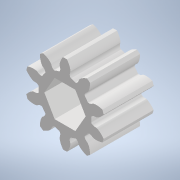
# Autodesk Inventor part: engranaje10
Saved by Autodesk Inventor 2022 (Build 260153000, 153)
## iProperties
Created: 2022-03-10
Part Number: engranaje10
Material: Generic
Document SubType Name: Modeling
Designer: katha
Density: 1 g/cm^3
Appearance: Default
Author: katha
Autodesk Inventor part; units mm, degrees
(part 1 of 2)
ref_plane "YZ Plane" through (0, 0, 0) normal (1, 0, 0) x (0, 1, 0)
ref_plane "XZ Plane" through (0, 0, 0) normal (0, 1, 0) x (-1, 0, 0)
ref_plane "XY Plane" through (0, 0, 0) normal (0, 0, 1) x (1, 0, 0)
sketch "Sketch1" plane through (0, 0, 0) normal (0, 0, 1) x (1, 0, 0)
  circle A0 centre (25, 0) radius 2
  circle A1 centre (25, 0) radius 2
  line L0 (21.2429, -4.5485) -> (21.2518, -4.404)
  line L1 (21.2518, -4.404) -> (21.266, -4.2669)
  line L2 (21.266, -4.2669) -> (21.2847, -4.1394)
  line L3 (21.2847, -4.1394) -> (21.3072, -4.0209)
  line L4 (21.3072, -4.0209) -> (21.3326, -3.9121)
  line L5 (21.3326, -3.9121) -> (21.3609, -3.8103)
  line L6 (21.3609, -3.8103) -> (21.3897, -3.7211)
  line L7 (21.3897, -3.7211) -> (21.4209, -3.6371)
  line L8 (21.4209, -3.6371) -> (21.4808, -3.5016)
  line L9 (21.4808, -3.5016) -> (21.5378, -3.3972)
  line L10 (21.5378, -3.3972) -> (21.5846, -3.3262)
  line L11 (21.5846, -3.3262) -> (21.6076, -3.2964)
  line L12 (21.6076, -3.2964) -> (21.7008, -3.2317)
  line L13 (21.7008, -3.2317) -> (21.7827, -3.1653)
  line L14 (21.7827, -3.1653) -> (21.8534, -3.098)
  line L15 (21.8534, -3.098) -> (21.9129, -3.0308)
  line L16 (21.9129, -3.0308) -> (21.9613, -2.9643)
  line L17 (21.9613, -2.9643) -> (21.9989, -2.8995)
  line L18 (21.9989, -2.8995) -> (22.026, -2.837)
  line L19 (22.026, -2.837) -> (22.0427, -2.7777)
  line L20 (22.0427, -2.7777) -> (22.0493, -2.7222)
  line L21 (22.0493, -2.7222) -> (22.0464, -2.6714)
  line L22 (22.0464, -2.6714) -> (22.0342, -2.626)
  line L23 (22.0342, -2.626) -> (22.0067, -2.5776)
  line L24 (22.0067, -2.5776) -> (21.911, -2.4618)
  line L25 (21.911, -2.4618) -> (21.8044, -2.3218)
  line L26 (21.8044, -2.3218) -> (21.7042, -2.1772)
  line L27 (21.7042, -2.1772) -> (21.6236, -2.0503)
  line L28 (21.6236, -2.0503) -> (21.5861, -2.0092)
  line L29 (21.5861, -2.0092) -> (21.5466, -1.9836)
  line L30 (21.5466, -1.9836) -> (21.4992, -1.9651)
  line L31 (21.4992, -1.9651) -> (21.4444, -1.9544)
  line L32 (21.4444, -1.9544) -> (21.3828, -1.9519)
  line L33 (21.3828, -1.9519) -> (21.3151, -1.9583)
  line L34 (21.3151, -1.9583) -> (21.2418, -1.974)
  line L35 (21.2418, -1.974) -> (21.1636, -1.9996)
  line L36 (21.1636, -1.9996) -> (21.0812, -2.0354)
  line L37 (21.0812, -2.0354) -> (20.9955, -2.0818)
  line L38 (20.9955, -2.0818) -> (20.907, -2.1392)
  line L39 (20.907, -2.1392) -> (20.8167, -2.2078)
  line L40 (20.8167, -2.2078) -> (20.7812, -2.2206)
  line L41 (20.7812, -2.2206) -> (20.6993, -2.2432)
  line L42 (20.6993, -2.2432) -> (20.5824, -2.2651)
  line L43 (20.5824, -2.2651) -> (20.4349, -2.2802)
  line L44 (20.4349, -2.2802) -> (20.3454, -2.2839)
  line L45 (20.3454, -2.2839) -> (20.2517, -2.2838)
  line L46 (20.2517, -2.2838) -> (20.1462, -2.2793)
  line L47 (20.1462, -2.2793) -> (20.0348, -2.2698)
  line L48 (20.0348, -2.2698) -> (19.9152, -2.2546)
  line L49 (19.9152, -2.2546) -> (19.7881, -2.2329)
  line L50 (19.7881, -2.2329) -> (19.6534, -2.2041)
  line L51 (19.6534, -2.2041) -> (19.5132, -2.1679)
  line L52 (19.5132, -2.1679) -> (19.3913, -2.1313)
  arc A2 (19.2098, -1.5727) -> (19.3913, -2.1313) centre (25, 0) ccw
  line L53 (19.2098, -1.5727) -> (19.2869, -1.4714)
  line L54 (19.2869, -1.4714) -> (19.379, -1.3597)
  line L55 (19.379, -1.3597) -> (19.4711, -1.2572)
  line L56 (19.4711, -1.2572) -> (19.5612, -1.165)
  line L57 (19.5612, -1.165) -> (19.649, -1.0823)
  line L58 (19.649, -1.0823) -> (19.7335, -1.0092)
  line L59 (19.7335, -1.0092) -> (19.8162, -0.9435)
  line L60 (19.8162, -0.9435) -> (19.892, -0.8884)
  line L61 (19.892, -0.8884) -> (19.9665, -0.8387)
  line L62 (19.9665, -0.8387) -> (20.0947, -0.7643)
  line L63 (20.0947, -0.7643) -> (20.2022, -0.7133)
  line L64 (20.2022, -0.7133) -> (20.2818, -0.6834)
  line L65 (20.2818, -0.6834) -> (20.3179, -0.6728)
  line L66 (20.3179, -0.6728) -> (20.4313, -0.6752)
  line L67 (20.4313, -0.6752) -> (20.5366, -0.6697)
  line L68 (20.5366, -0.6697) -> (20.6333, -0.6568)
  line L69 (20.6333, -0.6568) -> (20.721, -0.6373)
  line L70 (20.721, -0.6373) -> (20.7992, -0.6121)
  line L71 (20.7992, -0.6121) -> (20.8678, -0.5817)
  line L72 (20.8678, -0.5817) -> (20.9264, -0.5471)
  line L73 (20.9264, -0.5471) -> (20.9748, -0.5089)
  line L74 (20.9748, -0.5089) -> (21.0128, -0.468)
  line L75 (21.0128, -0.468) -> (21.0402, -0.4251)
  line L76 (21.0402, -0.4251) -> (21.0571, -0.3812)
  line L77 (21.0571, -0.3812) -> (21.0633, -0.3259)
  line L78 (21.0633, -0.3259) -> (21.0539, -0.1759)
  line L79 (21.0539, -0.1759) -> (21.05, 0)
  line L80 (21.05, 0) -> (21.0539, 0.1759)
  line L81 (21.0539, 0.1759) -> (21.0633, 0.3259)
  line L82 (21.0633, 0.3259) -> (21.0571, 0.3812)
  line L83 (21.0571, 0.3812) -> (21.0402, 0.4251)
  line L84 (21.0402, 0.4251) -> (21.0128, 0.468)
  line L85 (21.0128, 0.468) -> (20.9748, 0.5089)
  line L86 (20.9748, 0.5089) -> (20.9264, 0.5471)
  line L87 (20.9264, 0.5471) -> (20.8678, 0.5817)
  line L88 (20.8678, 0.5817) -> (20.7992, 0.6121)
  line L89 (20.7992, 0.6121) -> (20.721, 0.6373)
  line L90 (20.721, 0.6373) -> (20.6333, 0.6568)
  line L91 (20.6333, 0.6568) -> (20.5366, 0.6697)
  line L92 (20.5366, 0.6697) -> (20.4313, 0.6752)
  line L93 (20.4313, 0.6752) -> (20.3179, 0.6728)
  line L94 (20.3179, 0.6728) -> (20.2818, 0.6834)
  line L95 (20.2818, 0.6834) -> (20.2022, 0.7133)
  line L96 (20.2022, 0.7133) -> (20.0947, 0.7643)
  line L97 (20.0947, 0.7643) -> (19.9665, 0.8387)
  line L98 (19.9665, 0.8387) -> (19.892, 0.8884)
  line L99 (19.892, 0.8884) -> (19.8162, 0.9435)
  line L100 (19.8162, 0.9435) -> (19.7335, 1.0092)
  line L101 (19.7335, 1.0092) -> (19.649, 1.0823)
  line L102 (19.649, 1.0823) -> (19.5612, 1.165)
  line L103 (19.5612, 1.165) -> (19.4711, 1.2572)
  line L104 (19.4711, 1.2572) -> (19.379, 1.3597)
  line L105 (19.379, 1.3597) -> (19.2869, 1.4714)
  line L106 (19.2869, 1.4714) -> (19.2098, 1.5727)
  arc A3 (19.3913, 2.1312) -> (19.2098, 1.5727) centre (25, 0) ccw
  line L107 (19.3913, 2.1312) -> (19.5132, 2.1679)
  line L108 (19.5132, 2.1679) -> (19.6534, 2.2041)
  line L109 (19.6534, 2.2041) -> (19.7881, 2.2329)
  line L110 (19.7881, 2.2329) -> (19.9152, 2.2545)
  line L111 (19.9152, 2.2545) -> (20.0348, 2.2698)
  line L112 (20.0348, 2.2698) -> (20.1462, 2.2792)
  line L113 (20.1462, 2.2792) -> (20.2517, 2.2838)
  line L114 (20.2517, 2.2838) -> (20.3454, 2.2839)
  line L115 (20.3454, 2.2839) -> (20.4349, 2.2802)
  line L116 (20.4349, 2.2802) -> (20.5824, 2.2651)
  line L117 (20.5824, 2.2651) -> (20.6993, 2.2432)
  line L118 (20.6993, 2.2432) -> (20.7812, 2.2206)
  line L119 (20.7812, 2.2206) -> (20.8167, 2.2079)
  line L120 (20.8167, 2.2079) -> (20.907, 2.1393)
  line L121 (20.907, 2.1393) -> (20.9955, 2.0819)
  line L122 (20.9955, 2.0819) -> (21.0813, 2.0355)
  line L123 (21.0813, 2.0355) -> (21.1636, 1.9997)
  line L124 (21.1636, 1.9997) -> (21.2418, 1.9742)
  line L125 (21.2418, 1.9742) -> (21.3151, 1.9584)
  line L126 (21.3151, 1.9584) -> (21.3829, 1.952)
  line L127 (21.3829, 1.952) -> (21.4445, 1.9545)
  line L128 (21.4445, 1.9545) -> (21.4992, 1.9652)
  line L129 (21.4992, 1.9652) -> (21.5467, 1.9837)
  line L130 (21.5467, 1.9837) -> (21.5862, 2.0094)
  line L131 (21.5862, 2.0094) -> (21.6236, 2.0505)
  line L132 (21.6236, 2.0505) -> (21.7042, 2.1774)
  line L133 (21.7042, 2.1774) -> (21.8044, 2.3219)
  line L134 (21.8044, 2.3219) -> (21.911, 2.4619)
  line L135 (21.911, 2.4619) -> (22.0067, 2.5778)
  line L136 (22.0067, 2.5778) -> (22.0342, 2.6261)
  line L137 (22.0342, 2.6261) -> (22.0464, 2.6716)
  line L138 (22.0464, 2.6716) -> (22.0494, 2.7223)
  line L139 (22.0494, 2.7223) -> (22.0427, 2.7777)
  line L140 (22.0427, 2.7777) -> (22.026, 2.8371)
  line L141 (22.026, 2.8371) -> (21.999, 2.8995)
  line L142 (21.999, 2.8995) -> (21.9614, 2.9644)
  line L143 (21.9614, 2.9644) -> (21.9129, 3.0309)
  line L144 (21.9129, 3.0309) -> (21.8534, 3.0981)
  line L145 (21.8534, 3.0981) -> (21.7828, 3.1653)
  line L146 (21.7828, 3.1653) -> (21.7009, 3.2317)
  line L147 (21.7009, 3.2317) -> (21.6077, 3.2965)
  line L148 (21.6077, 3.2965) -> (21.5847, 3.3263)
  line L149 (21.5847, 3.3263) -> (21.5378, 3.3972)
  line L150 (21.5378, 3.3972) -> (21.4809, 3.5016)
  line L151 (21.4809, 3.5016) -> (21.4209, 3.6372)
  line L152 (21.4209, 3.6372) -> (21.3898, 3.7212)
  line L153 (21.3898, 3.7212) -> (21.3609, 3.8103)
  line L154 (21.3609, 3.8103) -> (21.3326, 3.9121)
  line L155 (21.3326, 3.9121) -> (21.3072, 4.0209)
  line L156 (21.3072, 4.0209) -> (21.2848, 4.1394)
  line L157 (21.2848, 4.1394) -> (21.2661, 4.2669)
  line L158 (21.2661, 4.2669) -> (21.2518, 4.404)
  line L159 (21.2518, 4.404) -> (21.2429, 4.5486)
  line L160 (21.2429, 4.5486) -> (21.2401, 4.6757)
  arc A4 (21.7156, 5.0212) -> (21.2401, 4.6757) centre (25, 0) ccw
  line L161 (21.7156, 5.0212) -> (21.8357, 4.9793)
  line L162 (21.8357, 4.9793) -> (21.9704, 4.9261)
  line L163 (21.9704, 4.9261) -> (22.0964, 4.8702)
  line L164 (22.0964, 4.8702) -> (22.2119, 4.813)
  line L165 (22.2119, 4.813) -> (22.3177, 4.7551)
  line L166 (22.3177, 4.7551) -> (22.4133, 4.6973)
  line L167 (22.4133, 4.6973) -> (22.5014, 4.6389)
  line L168 (22.5014, 4.6389) -> (22.5772, 4.584)
  line L169 (22.5772, 4.584) -> (22.6475, 4.5284)
  line L170 (22.6475, 4.5284) -> (22.7579, 4.4295)
  line L171 (22.7579, 4.4295) -> (22.8396, 4.3431)
  line L172 (22.8396, 4.3431) -> (22.8926, 4.2766)
  line L173 (22.8926, 4.2766) -> (22.9138, 4.2455)
  line L174 (22.9138, 4.2455) -> (22.9466, 4.1369)
  line L175 (22.9466, 4.1369) -> (22.9845, 4.0384)
  line L176 (22.9845, 4.0384) -> (23.0266, 3.9505)
  line L177 (23.0266, 3.9505) -> (23.0722, 3.8731)
  line L178 (23.0722, 3.8731) -> (23.1204, 3.8065)
  line L179 (23.1204, 3.8065) -> (23.1705, 3.7507)
  line L180 (23.1705, 3.7507) -> (23.2215, 3.7057)
  line L181 (23.2215, 3.7057) -> (23.2728, 3.6715)
  line L182 (23.2728, 3.6715) -> (23.3234, 3.648)
  line L183 (23.3234, 3.648) -> (23.3727, 3.6351)
  line L184 (23.3727, 3.6351) -> (23.4197, 3.6326)
  line L185 (23.4197, 3.6326) -> (23.4742, 3.6438)
  line L186 (23.4742, 3.6438) -> (23.6139, 3.6991)
  line L187 (23.6139, 3.6991) -> (23.78, 3.7572)
  line L188 (23.78, 3.7572) -> (23.9485, 3.8078)
  line L189 (23.9485, 3.8078) -> (24.094, 3.8453)
  line L190 (24.094, 3.8453) -> (24.1447, 3.8683)
  line L191 (24.1447, 3.8683) -> (24.1813, 3.8979)
  line L192 (24.1813, 3.8979) -> (24.2135, 3.9373)
  line L193 (24.2135, 3.9373) -> (24.2407, 3.9861)
  line L194 (24.2407, 3.9861) -> (24.262, 4.0439)
  line L195 (24.262, 4.0439) -> (24.2769, 4.1103)
  line L196 (24.2769, 4.1103) -> (24.2845, 4.1849)
  line L197 (24.2845, 4.1849) -> (24.2844, 4.2671)
  line L198 (24.2844, 4.2671) -> (24.2758, 4.3565)
  line L199 (24.2758, 4.3565) -> (24.2581, 4.4524)
  line L200 (24.2581, 4.4524) -> (24.2309, 4.5543)
  line L201 (24.2309, 4.5543) -> (24.1935, 4.6614)
  line L202 (24.1935, 4.6614) -> (24.1924, 4.6991)
  line L203 (24.1924, 4.6991) -> (24.1962, 4.784)
  line L204 (24.1962, 4.784) -> (24.2114, 4.902)
  line L205 (24.2114, 4.902) -> (24.2426, 5.0469)
  line L206 (24.2426, 5.0469) -> (24.2668, 5.1331)
  line L207 (24.2668, 5.1331) -> (24.2958, 5.2222)
  line L208 (24.2958, 5.2222) -> (24.3327, 5.3212)
  line L209 (24.3327, 5.3212) -> (24.3761, 5.4242)
  line L210 (24.3761, 5.4242) -> (24.4276, 5.5332)
  line L211 (24.4276, 5.5332) -> (24.4874, 5.6474)
  line L212 (24.4874, 5.6474) -> (24.5564, 5.7667)
  line L213 (24.5564, 5.7667) -> (24.6345, 5.8883)
  line L214 (24.6345, 5.8883) -> (24.7069, 5.9928)
  arc A5 (25.3, 5.9924) -> (24.7069, 5.9928) centre (25, 0) ccw
  line L215 (25.3, 5.9924) -> (25.3725, 5.8879)
  line L216 (25.3725, 5.8879) -> (25.4503, 5.7657)
  line L217 (25.4503, 5.7657) -> (25.5193, 5.6465)
  line L218 (25.5193, 5.6465) -> (25.5792, 5.5323)
  line L219 (25.5792, 5.5323) -> (25.6306, 5.4232)
  line L220 (25.6306, 5.4232) -> (25.6741, 5.3203)
  line L221 (25.6741, 5.3203) -> (25.711, 5.2213)
  line L222 (25.711, 5.2213) -> (25.7401, 5.1323)
  line L223 (25.7401, 5.1323) -> (25.7643, 5.046)
  line L224 (25.7643, 5.046) -> (25.7955, 4.9011)
  line L225 (25.7955, 4.9011) -> (25.8108, 4.7831)
  line L226 (25.8108, 4.7831) -> (25.8146, 4.6982)
  line L227 (25.8146, 4.6982) -> (25.8135, 4.6606)
  line L228 (25.8135, 4.6606) -> (25.7761, 4.5534)
  line L229 (25.7761, 4.5534) -> (25.7489, 4.4516)
  line L230 (25.7489, 4.4516) -> (25.7313, 4.3556)
  line L231 (25.7313, 4.3556) -> (25.7227, 4.2663)
  line L232 (25.7227, 4.2663) -> (25.7225, 4.184)
  line L233 (25.7225, 4.184) -> (25.7302, 4.1094)
  line L234 (25.7302, 4.1094) -> (25.7451, 4.043)
  line L235 (25.7451, 4.043) -> (25.7665, 3.9852)
  line L236 (25.7665, 3.9852) -> (25.7936, 3.9364)
  line L237 (25.7936, 3.9364) -> (25.8259, 3.8971)
  line L238 (25.8259, 3.8971) -> (25.8625, 3.8674)
  line L239 (25.8625, 3.8674) -> (25.9131, 3.8445)
  line L240 (25.9131, 3.8445) -> (26.0587, 3.807)
  line L241 (26.0587, 3.807) -> (26.2272, 3.7564)
  line L242 (26.2272, 3.7564) -> (26.3933, 3.6985)
  line L243 (26.3933, 3.6985) -> (26.5331, 3.6433)
  line L244 (26.5331, 3.6433) -> (26.5876, 3.6322)
  line L245 (26.5876, 3.6322) -> (26.6346, 3.6347)
  line L246 (26.6346, 3.6347) -> (26.6838, 3.6476)
  line L247 (26.6838, 3.6476) -> (26.7345, 3.6711)
  line L248 (26.7345, 3.6711) -> (26.7857, 3.7054)
  line L249 (26.7857, 3.7054) -> (26.8367, 3.7504)
  line L250 (26.8367, 3.7504) -> (26.8868, 3.8063)
  line L251 (26.8868, 3.8063) -> (26.9349, 3.873)
  line L252 (26.9349, 3.873) -> (26.9804, 3.9504)
  line L253 (26.9804, 3.9504) -> (27.0225, 4.0384)
  line L254 (27.0225, 4.0384) -> (27.0603, 4.1368)
  line L255 (27.0603, 4.1368) -> (27.0929, 4.2455)
  line L256 (27.0929, 4.2455) -> (27.1141, 4.2766)
  line L257 (27.1141, 4.2766) -> (27.1671, 4.3431)
  line L258 (27.1671, 4.3431) -> (27.2487, 4.4296)
  line L259 (27.2487, 4.4296) -> (27.359, 4.5286)
  line L260 (27.359, 4.5286) -> (27.4293, 4.5842)
  line L261 (27.4293, 4.5842) -> (27.5051, 4.6393)
  line L262 (27.5051, 4.6393) -> (27.5931, 4.6977)
  line L263 (27.5931, 4.6977) -> (27.6887, 4.7555)
  line L264 (27.6887, 4.7555) -> (27.7944, 4.8136)
  line L265 (27.7944, 4.8136) -> (27.9099, 4.8709)
  line L266 (27.9099, 4.8709) -> (28.0358, 4.9269)
  line L267 (28.0358, 4.9269) -> (28.1649, 4.9788)
  line L268 (28.1649, 4.9788) -> (28.2849, 5.0208)
  arc A6 (28.7599, 4.6757) -> (28.2849, 5.0208) centre (25, 0) ccw
  line L269 (28.7599, 4.6757) -> (28.7571, 4.5485)
  line L270 (28.7571, 4.5485) -> (28.7482, 4.4039)
  line L271 (28.7482, 4.4039) -> (28.734, 4.2669)
  line L272 (28.734, 4.2669) -> (28.7153, 4.1393)
  line L273 (28.7153, 4.1393) -> (28.6928, 4.0208)
  line L274 (28.6928, 4.0208) -> (28.6674, 3.912)
  line L275 (28.6674, 3.912) -> (28.6391, 3.8103)
  line L276 (28.6391, 3.8103) -> (28.6103, 3.7211)
  line L277 (28.6103, 3.7211) -> (28.5791, 3.6371)
  line L278 (28.5791, 3.6371) -> (28.5192, 3.5015)
  line L279 (28.5192, 3.5015) -> (28.4622, 3.3971)
  line L280 (28.4622, 3.3971) -> (28.4154, 3.3262)
  line L281 (28.4154, 3.3262) -> (28.3924, 3.2964)
  line L282 (28.3924, 3.2964) -> (28.2992, 3.2317)
  line L283 (28.2992, 3.2317) -> (28.2173, 3.1653)
  line L284 (28.2173, 3.1653) -> (28.1466, 3.098)
  line L285 (28.1466, 3.098) -> (28.0871, 3.0308)
  line L286 (28.0871, 3.0308) -> (28.0387, 2.9643)
  line L287 (28.0387, 2.9643) -> (28.0011, 2.8994)
  line L288 (28.0011, 2.8994) -> (27.974, 2.837)
  line L289 (27.974, 2.837) -> (27.9574, 2.7776)
  line L290 (27.9574, 2.7776) -> (27.9507, 2.7222)
  line L291 (27.9507, 2.7222) -> (27.9536, 2.6714)
  line L292 (27.9536, 2.6714) -> (27.9658, 2.6259)
  line L293 (27.9658, 2.6259) -> (27.9933, 2.5776)
  line L294 (27.9933, 2.5776) -> (28.089, 2.4617)
  line L295 (28.089, 2.4617) -> (28.1956, 2.3217)
  line L296 (28.1956, 2.3217) -> (28.2958, 2.1772)
  line L297 (28.2958, 2.1772) -> (28.3764, 2.0503)
  line L298 (28.3764, 2.0503) -> (28.4139, 2.0092)
  line L299 (28.4139, 2.0092) -> (28.4534, 1.9836)
  line L300 (28.4534, 1.9836) -> (28.5008, 1.9651)
  line L301 (28.5008, 1.9651) -> (28.5556, 1.9543)
  line L302 (28.5556, 1.9543) -> (28.6172, 1.9519)
  line L303 (28.6172, 1.9519) -> (28.6849, 1.9583)
  line L304 (28.6849, 1.9583) -> (28.7582, 1.974)
  line L305 (28.7582, 1.974) -> (28.8364, 1.9996)
  line L306 (28.8364, 1.9996) -> (28.9188, 2.0354)
  line L307 (28.9188, 2.0354) -> (29.0045, 2.0818)
  line L308 (29.0045, 2.0818) -> (29.093, 2.1392)
  line L309 (29.093, 2.1392) -> (29.1833, 2.2078)
  line L310 (29.1833, 2.2078) -> (29.2188, 2.2205)
  line L311 (29.2188, 2.2205) -> (29.3008, 2.2431)
  line L312 (29.3008, 2.2431) -> (29.4176, 2.265)
  line L313 (29.4176, 2.265) -> (29.5651, 2.2802)
  line L314 (29.5651, 2.2802) -> (29.6546, 2.2838)
  line L315 (29.6546, 2.2838) -> (29.7483, 2.2837)
  line L316 (29.7483, 2.2837) -> (29.8539, 2.2792)
  line L317 (29.8539, 2.2792) -> (29.9652, 2.2697)
  line L318 (29.9652, 2.2697) -> (30.0848, 2.2545)
  line L319 (30.0848, 2.2545) -> (30.2119, 2.2329)
  line L320 (30.2119, 2.2329) -> (30.3467, 2.2041)
  line L321 (30.3467, 2.2041) -> (30.4868, 2.1679)
  line L322 (30.4868, 2.1679) -> (30.6086, 2.1313)
  arc A7 (30.7902, 1.5727) -> (30.6086, 2.1313) centre (25, 0) ccw
  line L323 (30.7902, 1.5727) -> (30.7131, 1.4714)
  line L324 (30.7131, 1.4714) -> (30.6209, 1.3597)
  line L325 (30.6209, 1.3597) -> (30.5288, 1.2572)
  line L326 (30.5288, 1.2572) -> (30.4388, 1.165)
  line L327 (30.4388, 1.165) -> (30.3509, 1.0823)
  line L328 (30.3509, 1.0823) -> (30.2664, 1.0092)
  line L329 (30.2664, 1.0092) -> (30.1837, 0.9435)
  line L330 (30.1837, 0.9435) -> (30.108, 0.8884)
  line L331 (30.108, 0.8884) -> (30.0334, 0.8387)
  line L332 (30.0334, 0.8387) -> (29.9052, 0.7643)
  line L333 (29.9052, 0.7643) -> (29.7978, 0.7133)
  line L334 (29.7978, 0.7133) -> (29.7182, 0.6834)
  line L335 (29.7182, 0.6834) -> (29.6821, 0.6728)
  line L336 (29.6821, 0.6728) -> (29.5686, 0.6752)
  line L337 (29.5686, 0.6752) -> (29.4633, 0.6697)
  line L338 (29.4633, 0.6697) -> (29.3666, 0.6568)
  line L339 (29.3666, 0.6568) -> (29.279, 0.6373)
  line L340 (29.279, 0.6373) -> (29.2007, 0.6121)
  line L341 (29.2007, 0.6121) -> (29.1322, 0.5817)
  line L342 (29.1322, 0.5817) -> (29.0736, 0.547)
  line L343 (29.0736, 0.547) -> (29.0252, 0.5089)
  line L344 (29.0252, 0.5089) -> (28.9872, 0.4679)
  line L345 (28.9872, 0.4679) -> (28.9597, 0.4251)
  line L346 (28.9597, 0.4251) -> (28.9428, 0.3812)
  line L347 (28.9428, 0.3812) -> (28.9367, 0.3259)
  line L348 (28.9367, 0.3259) -> (28.9461, 0.1759)
  line L349 (28.9461, 0.1759) -> (28.95, 0)
  line L350 (28.95, 0) -> (28.9461, -0.1759)
  line L351 (28.9461, -0.1759) -> (28.9367, -0.3259)
  line L352 (28.9367, -0.3259) -> (28.9428, -0.3812)
  line L353 (28.9428, -0.3812) -> (28.9597, -0.4251)
  line L354 (28.9597, -0.4251) -> (28.9872, -0.468)
  line L355 (28.9872, -0.468) -> (29.0252, -0.5089)
  line L356 (29.0252, -0.5089) -> (29.0736, -0.5471)
  line L357 (29.0736, -0.5471) -> (29.1322, -0.5817)
  line L358 (29.1322, -0.5817) -> (29.2007, -0.6121)
  line L359 (29.2007, -0.6121) -> (29.279, -0.6374)
  line L360 (29.279, -0.6374) -> (29.3666, -0.6568)
  line L361 (29.3666, -0.6568) -> (29.4633, -0.6697)
  line L362 (29.4633, -0.6697) -> (29.5686, -0.6752)
  line L363 (29.5686, -0.6752) -> (29.6821, -0.6728)
  line L364 (29.6821, -0.6728) -> (29.7182, -0.6834)
  line L365 (29.7182, -0.6834) -> (29.7978, -0.7133)
  line L366 (29.7978, -0.7133) -> (29.9052, -0.7643)
  line L367 (29.9052, -0.7643) -> (30.0334, -0.8387)
  line L368 (30.0334, -0.8387) -> (30.108, -0.8884)
  line L369 (30.108, -0.8884) -> (30.1837, -0.9435)
  line L370 (30.1837, -0.9435) -> (30.2664, -1.0092)
  line L371 (30.2664, -1.0092) -> (30.3509, -1.0824)
  line L372 (30.3509, -1.0824) -> (30.4388, -1.165)
  line L373 (30.4388, -1.165) -> (30.5288, -1.2572)
  line L374 (30.5288, -1.2572) -> (30.6209, -1.3597)
  line L375 (30.6209, -1.3597) -> (30.7131, -1.4714)
  line L376 (30.7131, -1.4714) -> (30.7902, -1.5727)
  arc A8 (30.6087, -2.1311) -> (30.7902, -1.5727) centre (25, 0) ccw
  line L377 (30.6087, -2.1311) -> (30.4869, -2.1677)
  line L378 (30.4869, -2.1677) -> (30.3467, -2.2039)
  line L379 (30.3467, -2.2039) -> (30.2119, -2.2327)
  line L380 (30.2119, -2.2327) -> (30.0848, -2.2544)
  line L381 (30.0848, -2.2544) -> (29.9652, -2.2696)
  line L382 (29.9652, -2.2696) -> (29.8539, -2.2791)
  line L383 (29.8539, -2.2791) -> (29.7483, -2.2836)
  line L384 (29.7483, -2.2836) -> (29.6546, -2.2837)
  line L385 (29.6546, -2.2837) -> (29.5651, -2.2801)
  line L386 (29.5651, -2.2801) -> (29.4177, -2.265)
  line L387 (29.4177, -2.265) -> (29.3008, -2.243)
  line L388 (29.3008, -2.243) -> (29.2188, -2.2204)
  line L389 (29.2188, -2.2204) -> (29.1834, -2.2077)
  line L390 (29.1834, -2.2077) -> (29.093, -2.1391)
  line L391 (29.093, -2.1391) -> (29.0045, -2.0817)
  line L392 (29.0045, -2.0817) -> (28.9188, -2.0353)
  line L393 (28.9188, -2.0353) -> (28.8364, -1.9995)
  line L394 (28.8364, -1.9995) -> (28.7582, -1.974)
  line L395 (28.7582, -1.974) -> (28.6849, -1.9582)
  line L396 (28.6849, -1.9582) -> (28.6172, -1.9519)
  line L397 (28.6172, -1.9519) -> (28.5556, -1.9543)
  line L398 (28.5556, -1.9543) -> (28.5008, -1.9651)
  line L399 (28.5008, -1.9651) -> (28.4534, -1.9836)
  line L400 (28.4534, -1.9836) -> (28.4139, -2.0092)
  line L401 (28.4139, -2.0092) -> (28.3764, -2.0503)
  line L402 (28.3764, -2.0503) -> (28.2958, -2.1772)
  line L403 (28.2958, -2.1772) -> (28.1956, -2.3218)
  line L404 (28.1956, -2.3218) -> (28.0891, -2.4618)
  line L405 (28.0891, -2.4618) -> (27.9933, -2.5776)
  line L406 (27.9933, -2.5776) -> (27.9658, -2.626)
  line L407 (27.9658, -2.626) -> (27.9536, -2.6714)
  line L408 (27.9536, -2.6714) -> (27.9506, -2.7222)
  line L409 (27.9506, -2.7222) -> (27.9573, -2.7777)
  line L410 (27.9573, -2.7777) -> (27.974, -2.837)
  line L411 (27.974, -2.837) -> (28.001, -2.8995)
  line L412 (28.001, -2.8995) -> (28.0386, -2.9643)
  line L413 (28.0386, -2.9643) -> (28.0871, -3.0308)
  line L414 (28.0871, -3.0308) -> (28.1466, -3.098)
  line L415 (28.1466, -3.098) -> (28.2172, -3.1653)
  line L416 (28.2172, -3.1653) -> (28.2991, -3.2317)
  line L417 (28.2991, -3.2317) -> (28.3923, -3.2964)
  line L418 (28.3923, -3.2964) -> (28.4154, -3.3262)
  line L419 (28.4154, -3.3262) -> (28.4622, -3.3971)
  line L420 (28.4622, -3.3971) -> (28.5192, -3.5016)
  line L421 (28.5192, -3.5016) -> (28.5791, -3.6371)
  line L422 (28.5791, -3.6371) -> (28.6102, -3.7211)
  line L423 (28.6102, -3.7211) -> (28.6391, -3.8103)
  line L424 (28.6391, -3.8103) -> (28.6674, -3.912)
  line L425 (28.6674, -3.912) -> (28.6928, -4.0208)
  line L426 (28.6928, -4.0208) -> (28.7153, -4.1393)
  line L427 (28.7153, -4.1393) -> (28.734, -4.2669)
  line L428 (28.734, -4.2669) -> (28.7482, -4.4039)
  line L429 (28.7482, -4.4039) -> (28.7571, -4.5485)
  line L430 (28.7571, -4.5485) -> (28.7599, -4.6757)
  arc A9 (28.2849, -5.0208) -> (28.7599, -4.6757) centre (25, 0) ccw
  line L431 (28.2849, -5.0208) -> (28.1648, -4.9789)
  line L432 (28.1648, -4.9789) -> (28.0301, -4.9258)
  line L433 (28.0301, -4.9258) -> (27.9042, -4.8699)
  line L434 (27.9042, -4.8699) -> (27.7886, -4.8127)
  line L435 (27.7886, -4.8127) -> (27.6829, -4.7547)
  line L436 (27.6829, -4.7547) -> (27.5872, -4.697)
  line L437 (27.5872, -4.697) -> (27.4992, -4.6386)
  line L438 (27.4992, -4.6386) -> (27.4233, -4.5836)
  line L439 (27.4233, -4.5836) -> (27.353, -4.528)
  line L440 (27.353, -4.528) -> (27.2426, -4.4291)
  line L441 (27.2426, -4.4291) -> (27.1609, -4.3427)
  line L442 (27.1609, -4.3427) -> (27.1079, -4.2763)
  line L443 (27.1079, -4.2763) -> (27.0867, -4.2451)
  line L444 (27.0867, -4.2451) -> (27.0539, -4.1365)
  line L445 (27.0539, -4.1365) -> (27.0161, -4.0381)
  line L446 (27.0161, -4.0381) -> (26.974, -3.9501)
  line L447 (26.974, -3.9501) -> (26.9284, -3.8728)
  line L448 (26.9284, -3.8728) -> (26.8802, -3.8062)
  line L449 (26.8802, -3.8062) -> (26.8301, -3.7503)
  line L450 (26.8301, -3.7503) -> (26.779, -3.7053)
  line L451 (26.779, -3.7053) -> (26.7278, -3.6711)
  line L452 (26.7278, -3.6711) -> (26.6771, -3.6476)
  line L453 (26.6771, -3.6476) -> (26.6279, -3.6347)
  line L454 (26.6279, -3.6347) -> (26.5809, -3.6323)
  line L455 (26.5809, -3.6323) -> (26.5264, -3.6435)
  line L456 (26.5264, -3.6435) -> (26.3866, -3.6988)
  line L457 (26.3866, -3.6988) -> (26.2206, -3.7568)
  line L458 (26.2206, -3.7568) -> (26.0521, -3.8075)
  line L459 (26.0521, -3.8075) -> (25.9065, -3.8449)
  line L460 (25.9065, -3.8449) -> (25.8559, -3.8679)
  line L461 (25.8559, -3.8679) -> (25.8193, -3.8976)
  line L462 (25.8193, -3.8976) -> (25.7871, -3.9369)
  line L463 (25.7871, -3.9369) -> (25.7599, -3.9857)
  line L464 (25.7599, -3.9857) -> (25.7385, -4.0435)
  line L465 (25.7385, -4.0435) -> (25.7237, -4.11)
  line L466 (25.7237, -4.11) -> (25.716, -4.1846)
  line L467 (25.716, -4.1846) -> (25.7162, -4.2668)
  line L468 (25.7162, -4.2668) -> (25.7248, -4.3562)
  line L469 (25.7248, -4.3562) -> (25.7424, -4.4521)
  line L470 (25.7424, -4.4521) -> (25.7697, -4.5539)
  line L471 (25.7697, -4.5539) -> (25.8071, -4.6611)
  line L472 (25.8071, -4.6611) -> (25.8082, -4.6987)
  line L473 (25.8082, -4.6987) -> (25.8044, -4.7837)
  line L474 (25.8044, -4.7837) -> (25.7891, -4.9016)
  line L475 (25.7891, -4.9016) -> (25.758, -5.0465)
  line L476 (25.758, -5.0465) -> (25.7338, -5.1328)
  line L477 (25.7338, -5.1328) -> (25.7047, -5.2219)
  line L478 (25.7047, -5.2219) -> (25.6678, -5.3209)
  line L479 (25.6678, -5.3209) -> (25.6244, -5.4238)
  line L480 (25.6244, -5.4238) -> (25.573, -5.5329)
  line L481 (25.573, -5.5329) -> (25.5132, -5.6471)
  line L482 (25.5132, -5.6471) -> (25.4441, -5.7663)
  line L483 (25.4441, -5.7663) -> (25.3659, -5.8882)
  line L484 (25.3659, -5.8882) -> (25.2934, -5.9928)
  arc A10 (24.7065, -5.9928) -> (25.2934, -5.9928) centre (25, 0) ccw
  line L485 (24.7065, -5.9928) -> (24.634, -5.8882)
  line L486 (24.634, -5.8882) -> (24.5563, -5.7661)
  line L487 (24.5563, -5.7661) -> (24.4872, -5.6468)
  line L488 (24.4872, -5.6468) -> (24.4273, -5.5326)
  line L489 (24.4273, -5.5326) -> (24.3759, -5.4236)
  line L490 (24.3759, -5.4236) -> (24.3325, -5.3206)
  line L491 (24.3325, -5.3206) -> (24.2955, -5.2217)
  line L492 (24.2955, -5.2217) -> (24.2665, -5.1326)
  line L493 (24.2665, -5.1326) -> (24.2423, -5.0463)
  line L494 (24.2423, -5.0463) -> (24.2111, -4.9014)
  line L495 (24.2111, -4.9014) -> (24.1958, -4.7835)
  line L496 (24.1958, -4.7835) -> (24.1919, -4.6986)
  line L497 (24.1919, -4.6986) -> (24.1931, -4.6609)
  line L498 (24.1931, -4.6609) -> (24.2304, -4.5538)
  line L499 (24.2304, -4.5538) -> (24.2576, -4.4519)
  line L500 (24.2576, -4.4519) -> (24.2752, -4.356)
  line L501 (24.2752, -4.356) -> (24.2838, -4.2666)
  line L502 (24.2838, -4.2666) -> (24.284, -4.1843)
  line L503 (24.284, -4.1843) -> (24.2763, -4.1098)
  line L504 (24.2763, -4.1098) -> (24.2614, -4.0433)
  line L505 (24.2614, -4.0433) -> (24.24, -3.9855)
  line L506 (24.24, -3.9855) -> (24.2129, -3.9368)
  line L507 (24.2129, -3.9368) -> (24.1806, -3.8974)
  line L508 (24.1806, -3.8974) -> (24.144, -3.8677)
  line L509 (24.144, -3.8677) -> (24.0934, -3.8448)
  line L510 (24.0934, -3.8448) -> (23.9478, -3.8074)
  line L511 (23.9478, -3.8074) -> (23.7793, -3.7568)
  line L512 (23.7793, -3.7568) -> (23.6132, -3.6988)
  line L513 (23.6132, -3.6988) -> (23.4734, -3.6436)
  line L514 (23.4734, -3.6436) -> (23.4189, -3.6325)
  line L515 (23.4189, -3.6325) -> (23.3719, -3.635)
  line L516 (23.3719, -3.635) -> (23.3227, -3.6479)
  line L517 (23.3227, -3.6479) -> (23.272, -3.6715)
  line L518 (23.272, -3.6715) -> (23.2208, -3.7057)
  line L519 (23.2208, -3.7057) -> (23.1698, -3.7508)
  line L520 (23.1698, -3.7508) -> (23.1198, -3.8066)
  line L521 (23.1198, -3.8066) -> (23.0716, -3.8733)
  line L522 (23.0716, -3.8733) -> (23.0261, -3.9507)
  line L523 (23.0261, -3.9507) -> (22.984, -4.0387)
  line L524 (22.984, -4.0387) -> (22.9463, -4.1371)
  line L525 (22.9463, -4.1371) -> (22.9136, -4.2458)
  line L526 (22.9136, -4.2458) -> (22.8924, -4.2769)
  line L527 (22.8924, -4.2769) -> (22.8394, -4.3434)
  line L528 (22.8394, -4.3434) -> (22.7578, -4.4299)
  line L529 (22.7578, -4.4299) -> (22.6475, -4.5289)
  line L530 (22.6475, -4.5289) -> (22.5773, -4.5845)
  line L531 (22.5773, -4.5845) -> (22.5014, -4.6396)
  line L532 (22.5014, -4.6396) -> (22.4134, -4.698)
  line L533 (22.4134, -4.698) -> (22.3178, -4.7559)
  line L534 (22.3178, -4.7559) -> (22.2121, -4.8139)
  line L535 (22.2121, -4.8139) -> (22.0967, -4.8712)
  line L536 (22.0967, -4.8712) -> (21.9707, -4.9272)
  line L537 (21.9707, -4.9272) -> (21.8364, -4.9813)
  line L538 (21.8364, -4.9813) -> (21.7179, -5.0227)
  arc A11 (21.2401, -4.6757) -> (21.7179, -5.0227) centre (25, 0) ccw
  line L539 (21.2401, -4.6757) -> (21.2429, -4.5485)
  line L540 (21.2429, -4.5485) -> (21.2518, -4.404)
  line L541 (21.2518, -4.404) -> (21.266, -4.2669)
  line L542 (21.266, -4.2669) -> (21.2847, -4.1394)
  line L543 (21.2847, -4.1394) -> (21.3072, -4.0209)
  line L544 (21.3072, -4.0209) -> (21.3326, -3.9121)
  line L545 (21.3326, -3.9121) -> (21.3609, -3.8103)
  line L546 (21.3609, -3.8103) -> (21.3897, -3.7211)
  line L547 (21.3897, -3.7211) -> (21.4209, -3.6371)
  line L548 (21.4209, -3.6371) -> (21.4808, -3.5016)
  line L549 (21.4808, -3.5016) -> (21.5378, -3.3972)
  line L550 (21.5378, -3.3972) -> (21.5846, -3.3262)
  line L551 (21.5846, -3.3262) -> (21.6076, -3.2964)
  line L552 (21.6076, -3.2964) -> (21.7008, -3.2317)
  line L553 (21.7008, -3.2317) -> (21.7827, -3.1653)
  line L554 (21.7827, -3.1653) -> (21.8534, -3.098)
  line L555 (21.8534, -3.098) -> (21.9129, -3.0308)
  line L556 (21.9129, -3.0308) -> (21.9613, -2.9643)
  line L557 (21.9613, -2.9643) -> (21.9989, -2.8995)
  line L558 (21.9989, -2.8995) -> (22.026, -2.837)
  line L559 (22.026, -2.837) -> (22.0427, -2.7777)
  line L560 (22.0427, -2.7777) -> (22.0493, -2.7222)
  line L561 (22.0493, -2.7222) -> (22.0464, -2.6714)
  line L562 (22.0464, -2.6714) -> (22.0342, -2.626)
  line L563 (22.0342, -2.626) -> (22.0067, -2.5776)
  line L564 (22.0067, -2.5776) -> (21.911, -2.4618)
  line L565 (21.911, -2.4618) -> (21.8044, -2.3218)
  line L566 (21.8044, -2.3218) -> (21.7042, -2.1772)
  line L567 (21.7042, -2.1772) -> (21.6236, -2.0503)
  line L568 (21.6236, -2.0503) -> (21.5861, -2.0092)
  line L569 (21.5861, -2.0092) -> (21.5466, -1.9836)
  line L570 (21.5466, -1.9836) -> (21.4992, -1.9651)
  line L571 (21.4992, -1.9651) -> (21.4444, -1.9544)
  line L572 (21.4444, -1.9544) -> (21.3828, -1.9519)
  line L573 (21.3828, -1.9519) -> (21.3151, -1.9583)
  line L574 (21.3151, -1.9583) -> (21.2418, -1.974)
  line L575 (21.2418, -1.974) -> (21.1636, -1.9996)
  line L576 (21.1636, -1.9996) -> (21.0812, -2.0354)
  line L577 (21.0812, -2.0354) -> (20.9955, -2.0818)
  line L578 (20.9955, -2.0818) -> (20.907, -2.1392)
  line L579 (20.907, -2.1392) -> (20.8167, -2.2078)
  line L580 (20.8167, -2.2078) -> (20.7812, -2.2206)
  line L581 (20.7812, -2.2206) -> (20.6993, -2.2432)
  line L582 (20.6993, -2.2432) -> (20.5824, -2.2651)
  line L583 (20.5824, -2.2651) -> (20.4349, -2.2802)
  line L584 (20.4349, -2.2802) -> (20.3454, -2.2839)
  line L585 (20.3454, -2.2839) -> (20.2517, -2.2838)
  line L586 (20.2517, -2.2838) -> (20.1462, -2.2793)
  line L587 (20.1462, -2.2793) -> (20.0348, -2.2698)
  line L588 (20.0348, -2.2698) -> (19.9152, -2.2546)
  line L589 (19.9152, -2.2546) -> (19.7881, -2.2329)
  line L590 (19.7881, -2.2329) -> (19.6534, -2.2041)
  line L591 (19.6534, -2.2041) -> (19.5132, -2.1679)
  line L592 (19.5132, -2.1679) -> (19.3913, -2.1313)
  arc A12 (19.2098, -1.5727) -> (19.3913, -2.1313) centre (25, 0) ccw
  line L593 (19.2098, -1.5727) -> (19.2869, -1.4714)
  line L594 (19.2869, -1.4714) -> (19.379, -1.3597)
  line L595 (19.379, -1.3597) -> (19.4711, -1.2572)
  line L596 (19.4711, -1.2572) -> (19.5612, -1.165)
  line L597 (19.5612, -1.165) -> (19.649, -1.0823)
  line L598 (19.649, -1.0823) -> (19.7335, -1.0092)
  line L599 (19.7335, -1.0092) -> (19.8162, -0.9435)
  line L600 (19.8162, -0.9435) -> (19.892, -0.8884)
  line L601 (19.892, -0.8884) -> (19.9665, -0.8387)
  line L602 (19.9665, -0.8387) -> (20.0947, -0.7643)
  line L603 (20.0947, -0.7643) -> (20.2022, -0.7133)
  line L604 (20.2022, -0.7133) -> (20.2818, -0.6834)
  line L605 (20.2818, -0.6834) -> (20.3179, -0.6728)
  line L606 (20.3179, -0.6728) -> (20.4313, -0.6752)
  line L607 (20.4313, -0.6752) -> (20.5366, -0.6697)
  line L608 (20.5366, -0.6697) -> (20.6333, -0.6568)
  line L609 (20.6333, -0.6568) -> (20.721, -0.6373)
  line L610 (20.721, -0.6373) -> (20.7992, -0.6121)
  line L611 (20.7992, -0.6121) -> (20.8678, -0.5817)
  line L612 (20.8678, -0.5817) -> (20.9264, -0.5471)
  line L613 (20.9264, -0.5471) -> (20.9748, -0.5089)
  line L614 (20.9748, -0.5089) -> (21.0128, -0.468)
  line L615 (21.0128, -0.468) -> (21.0402, -0.4251)
  line L616 (21.0402, -0.4251) -> (21.0571, -0.3812)
  line L617 (21.0571, -0.3812) -> (21.0633, -0.3259)
  line L618 (21.0633, -0.3259) -> (21.0539, -0.1759)
  line L619 (21.0539, -0.1759) -> (21.05, 0)
  line L620 (21.05, 0) -> (21.0539, 0.1759)
  line L621 (21.0539, 0.1759) -> (21.0633, 0.3259)
  line L622 (21.0633, 0.3259) -> (21.0571, 0.3812)
  line L623 (21.0571, 0.3812) -> (21.0402, 0.4251)
  line L624 (21.0402, 0.4251) -> (21.0128, 0.468)
  line L625 (21.0128, 0.468) -> (20.9748, 0.5089)
  line L626 (20.9748, 0.5089) -> (20.9264, 0.5471)
  line L627 (20.9264, 0.5471) -> (20.8678, 0.5817)
  line L628 (20.8678, 0.5817) -> (20.7992, 0.6121)
  line L629 (20.7992, 0.6121) -> (20.721, 0.6373)
  line L630 (20.721, 0.6373) -> (20.6333, 0.6568)
  line L631 (20.6333, 0.6568) -> (20.5366, 0.6697)
  line L632 (20.5366, 0.6697) -> (20.4313, 0.6752)
  line L633 (20.4313, 0.6752) -> (20.3179, 0.6728)
  line L634 (20.3179, 0.6728) -> (20.2818, 0.6834)
  line L635 (20.2818, 0.6834) -> (20.2022, 0.7133)
  line L636 (20.2022, 0.7133) -> (20.0947, 0.7643)
  line L637 (20.0947, 0.7643) -> (19.9665, 0.8387)
  line L638 (19.9665, 0.8387) -> (19.892, 0.8884)
  line L639 (19.892, 0.8884) -> (19.8162, 0.9435)
  line L640 (19.8162, 0.9435) -> (19.7335, 1.0092)
  line L641 (19.7335, 1.0092) -> (19.649, 1.0823)
  line L642 (19.649, 1.0823) -> (19.5612, 1.165)
  line L643 (19.5612, 1.165) -> (19.4711, 1.2572)
  line L644 (19.4711, 1.2572) -> (19.379, 1.3597)
  line L645 (19.379, 1.3597) -> (19.2869, 1.4714)
  line L646 (19.2869, 1.4714) -> (19.2098, 1.5727)
  arc A13 (19.3913, 2.1312) -> (19.2098, 1.5727) centre (25, 0) ccw
  line L647 (19.3913, 2.1312) -> (19.5132, 2.1679)
  line L648 (19.5132, 2.1679) -> (19.6534, 2.2041)
  line L649 (19.6534, 2.2041) -> (19.7881, 2.2329)
  line L650 (19.7881, 2.2329) -> (19.9152, 2.2545)
  line L651 (19.9152, 2.2545) -> (20.0348, 2.2698)
  line L652 (20.0348, 2.2698) -> (20.1462, 2.2792)
  line L653 (20.1462, 2.2792) -> (20.2517, 2.2838)
  line L654 (20.2517, 2.2838) -> (20.3454, 2.2839)
  line L655 (20.3454, 2.2839) -> (20.4349, 2.2802)
  line L656 (20.4349, 2.2802) -> (20.5824, 2.2651)
  line L657 (20.5824, 2.2651) -> (20.6993, 2.2432)
  line L658 (20.6993, 2.2432) -> (20.7812, 2.2206)
  line L659 (20.7812, 2.2206) -> (20.8167, 2.2079)
  line L660 (20.8167, 2.2079) -> (20.907, 2.1393)
  line L661 (20.907, 2.1393) -> (20.9955, 2.0819)
  line L662 (20.9955, 2.0819) -> (21.0813, 2.0355)
  line L663 (21.0813, 2.0355) -> (21.1636, 1.9997)
  line L664 (21.1636, 1.9997) -> (21.2418, 1.9742)
  line L665 (21.2418, 1.9742) -> (21.3151, 1.9584)
  line L666 (21.3151, 1.9584) -> (21.3829, 1.952)
  line L667 (21.3829, 1.952) -> (21.4445, 1.9545)
  line L668 (21.4445, 1.9545) -> (21.4992, 1.9652)
  line L669 (21.4992, 1.9652) -> (21.5467, 1.9837)
  line L670 (21.5467, 1.9837) -> (21.5862, 2.0094)
  line L671 (21.5862, 2.0094) -> (21.6236, 2.0505)
  line L672 (21.6236, 2.0505) -> (21.7042, 2.1774)
  line L673 (21.7042, 2.1774) -> (21.8044, 2.3219)
  line L674 (21.8044, 2.3219) -> (21.911, 2.4619)
  line L675 (21.911, 2.4619) -> (22.0067, 2.5778)
  line L676 (22.0067, 2.5778) -> (22.0342, 2.6261)
  line L677 (22.0342, 2.6261) -> (22.0464, 2.6716)
  line L678 (22.0464, 2.6716) -> (22.0494, 2.7223)
  line L679 (22.0494, 2.7223) -> (22.0427, 2.7777)
  line L680 (22.0427, 2.7777) -> (22.026, 2.8371)
  line L681 (22.026, 2.8371) -> (21.999, 2.8995)
  line L682 (21.999, 2.8995) -> (21.9614, 2.9644)
  line L683 (21.9614, 2.9644) -> (21.9129, 3.0309)
  line L684 (21.9129, 3.0309) -> (21.8534, 3.0981)
  line L685 (21.8534, 3.0981) -> (21.7828, 3.1653)
  line L686 (21.7828, 3.1653) -> (21.7009, 3.2317)
  line L687 (21.7009, 3.2317) -> (21.6077, 3.2965)
  line L688 (21.6077, 3.2965) -> (21.5847, 3.3263)
  line L689 (21.5847, 3.3263) -> (21.5378, 3.3972)
  line L690 (21.5378, 3.3972) -> (21.4809, 3.5016)
  line L691 (21.4809, 3.5016) -> (21.4209, 3.6372)
  line L692 (21.4209, 3.6372) -> (21.3898, 3.7212)
  line L693 (21.3898, 3.7212) -> (21.3609, 3.8103)
  line L694 (21.3609, 3.8103) -> (21.3326, 3.9121)
  line L695 (21.3326, 3.9121) -> (21.3072, 4.0209)
  line L696 (21.3072, 4.0209) -> (21.2848, 4.1394)
  line L697 (21.2848, 4.1394) -> (21.2661, 4.2669)
  line L698 (21.2661, 4.2669) -> (21.2518, 4.404)
  line L699 (21.2518, 4.404) -> (21.2429, 4.5486)
  line L700 (21.2429, 4.5486) -> (21.2401, 4.6757)
  arc A14 (21.7156, 5.0212) -> (21.2401, 4.6757) centre (25, 0) ccw
  line L701 (21.7156, 5.0212) -> (21.8357, 4.9793)
  line L702 (21.8357, 4.9793) -> (21.9704, 4.9261)
  line L703 (21.9704, 4.9261) -> (22.0964, 4.8702)
  line L704 (22.0964, 4.8702) -> (22.2119, 4.813)
  line L705 (22.2119, 4.813) -> (22.3177, 4.7551)
  line L706 (22.3177, 4.7551) -> (22.4133, 4.6973)
  line L707 (22.4133, 4.6973) -> (22.5014, 4.6389)
  line L708 (22.5014, 4.6389) -> (22.5772, 4.584)
  line L709 (22.5772, 4.584) -> (22.6475, 4.5284)
  line L710 (22.6475, 4.5284) -> (22.7579, 4.4295)
  line L711 (22.7579, 4.4295) -> (22.8396, 4.3431)
  line L712 (22.8396, 4.3431) -> (22.8926, 4.2766)
  line L713 (22.8926, 4.2766) -> (22.9138, 4.2455)
  line L714 (22.9138, 4.2455) -> (22.9466, 4.1369)
  line L715 (22.9466, 4.1369) -> (22.9845, 4.0384)
  line L716 (22.9845, 4.0384) -> (23.0266, 3.9505)
  line L717 (23.0266, 3.9505) -> (23.0722, 3.8731)
  line L718 (23.0722, 3.8731) -> (23.1204, 3.8065)
  line L719 (23.1204, 3.8065) -> (23.1705, 3.7507)
  line L720 (23.1705, 3.7507) -> (23.2215, 3.7057)
  line L721 (23.2215, 3.7057) -> (23.2728, 3.6715)
  line L722 (23.2728, 3.6715) -> (23.3234, 3.648)
  line L723 (23.3234, 3.648) -> (23.3727, 3.6351)
  line L724 (23.3727, 3.6351) -> (23.4197, 3.6326)
  line L725 (23.4197, 3.6326) -> (23.4742, 3.6438)
  line L726 (23.4742, 3.6438) -> (23.6139, 3.6991)
  line L727 (23.6139, 3.6991) -> (23.78, 3.7572)
  line L728 (23.78, 3.7572) -> (23.9485, 3.8078)
  line L729 (23.9485, 3.8078) -> (24.094, 3.8453)
  line L730 (24.094, 3.8453) -> (24.1447, 3.8683)
  line L731 (24.1447, 3.8683) -> (24.1813, 3.8979)
  line L732 (24.1813, 3.8979) -> (24.2135, 3.9373)
  line L733 (24.2135, 3.9373) -> (24.2407, 3.9861)
  line L734 (24.2407, 3.9861) -> (24.262, 4.0439)
  line L735 (24.262, 4.0439) -> (24.2769, 4.1103)
  line L736 (24.2769, 4.1103) -> (24.2845, 4.1849)
  line L737 (24.2845, 4.1849) -> (24.2844, 4.2671)
  line L738 (24.2844, 4.2671) -> (24.2758, 4.3565)
  line L739 (24.2758, 4.3565) -> (24.2581, 4.4524)
  line L740 (24.2581, 4.4524) -> (24.2309, 4.5543)
  line L741 (24.2309, 4.5543) -> (24.1935, 4.6614)
  line L742 (24.1935, 4.6614) -> (24.1924, 4.6991)
  line L743 (24.1924, 4.6991) -> (24.1962, 4.784)
  line L744 (24.1962, 4.784) -> (24.2114, 4.902)
  line L745 (24.2114, 4.902) -> (24.2426, 5.0469)
  line L746 (24.2426, 5.0469) -> (24.2668, 5.1331)
  line L747 (24.2668, 5.1331) -> (24.2958, 5.2222)
  line L748 (24.2958, 5.2222) -> (24.3327, 5.3212)
  line L749 (24.3327, 5.3212) -> (24.3761, 5.4242)
  line L750 (24.3761, 5.4242) -> (24.4276, 5.5332)
  line L751 (24.4276, 5.5332) -> (24.4874, 5.6474)
  line L752 (24.4874, 5.6474) -> (24.5564, 5.7667)
  line L753 (24.5564, 5.7667) -> (24.6345, 5.8883)
  line L754 (24.6345, 5.8883) -> (24.7069, 5.9928)
  arc A15 (25.3, 5.9924) -> (24.7069, 5.9928) centre (25, 0) ccw
  line L755 (25.3, 5.9924) -> (25.3725, 5.8879)
  line L756 (25.3725, 5.8879) -> (25.4503, 5.7657)
  line L757 (25.4503, 5.7657) -> (25.5193, 5.6465)
  line L758 (25.5193, 5.6465) -> (25.5792, 5.5323)
  line L759 (25.5792, 5.5323) -> (25.6306, 5.4232)
  line L760 (25.6306, 5.4232) -> (25.6741, 5.3203)
  line L761 (25.6741, 5.3203) -> (25.711, 5.2213)
  line L762 (25.711, 5.2213) -> (25.7401, 5.1323)
  line L763 (25.7401, 5.1323) -> (25.7643, 5.046)
  line L764 (25.7643, 5.046) -> (25.7955, 4.9011)
  line L765 (25.7955, 4.9011) -> (25.8108, 4.7831)
  line L766 (25.8108, 4.7831) -> (25.8146, 4.6982)
  line L767 (25.8146, 4.6982) -> (25.8135, 4.6606)
  line L768 (25.8135, 4.6606) -> (25.7761, 4.5534)
  line L769 (25.7761, 4.5534) -> (25.7489, 4.4516)
  line L770 (25.7489, 4.4516) -> (25.7313, 4.3556)
  line L771 (25.7313, 4.3556) -> (25.7227, 4.2663)
  line L772 (25.7227, 4.2663) -> (25.7225, 4.184)
  line L773 (25.7225, 4.184) -> (25.7302, 4.1094)
  line L774 (25.7302, 4.1094) -> (25.7451, 4.043)
  line L775 (25.7451, 4.043) -> (25.7665, 3.9852)
  line L776 (25.7665, 3.9852) -> (25.7936, 3.9364)
  line L777 (25.7936, 3.9364) -> (25.8259, 3.8971)
  line L778 (25.8259, 3.8971) -> (25.8625, 3.8674)
  line L779 (25.8625, 3.8674) -> (25.9131, 3.8445)
  line L780 (25.9131, 3.8445) -> (26.0587, 3.807)
  line L781 (26.0587, 3.807) -> (26.2272, 3.7564)
  line L782 (26.2272, 3.7564) -> (26.3933, 3.6985)
  line L783 (26.3933, 3.6985) -> (26.5331, 3.6433)
  line L784 (26.5331, 3.6433) -> (26.5876, 3.6322)
  line L785 (26.5876, 3.6322) -> (26.6346, 3.6347)
  line L786 (26.6346, 3.6347) -> (26.6838, 3.6476)
  line L787 (26.6838, 3.6476) -> (26.7345, 3.6711)
  line L788 (26.7345, 3.6711) -> (26.7857, 3.7054)
  line L789 (26.7857, 3.7054) -> (26.8367, 3.7504)
  line L790 (26.8367, 3.7504) -> (26.8868, 3.8063)
  line L791 (26.8868, 3.8063) -> (26.9349, 3.873)
  line L792 (26.9349, 3.873) -> (26.9804, 3.9504)
  line L793 (26.9804, 3.9504) -> (27.0225, 4.0384)
  line L794 (27.0225, 4.0384) -> (27.0603, 4.1368)
  line L795 (27.0603, 4.1368) -> (27.0929, 4.2455)
  line L796 (27.0929, 4.2455) -> (27.1141, 4.2766)
  line L797 (27.1141, 4.2766) -> (27.1671, 4.3431)
  line L798 (27.1671, 4.3431) -> (27.2487, 4.4296)
  line L799 (27.2487, 4.4296) -> (27.359, 4.5286)
  line L800 (27.359, 4.5286) -> (27.4293, 4.5842)
  line L801 (27.4293, 4.5842) -> (27.5051, 4.6393)
  line L802 (27.5051, 4.6393) -> (27.5931, 4.6977)
  line L803 (27.5931, 4.6977) -> (27.6887, 4.7555)
  line L804 (27.6887, 4.7555) -> (27.7944, 4.8136)
  line L805 (27.7944, 4.8136) -> (27.9099, 4.8709)
  line L806 (27.9099, 4.8709) -> (28.0358, 4.9269)
  line L807 (28.0358, 4.9269) -> (28.1649, 4.9788)
  line L808 (28.1649, 4.9788) -> (28.2849, 5.0208)
  arc A16 (28.7599, 4.6757) -> (28.2849, 5.0208) centre (25, 0) ccw
  line L809 (28.7599, 4.6757) -> (28.7571, 4.5485)
  line L810 (28.7571, 4.5485) -> (28.7482, 4.4039)
  line L811 (28.7482, 4.4039) -> (28.734, 4.2669)
  line L812 (28.734, 4.2669) -> (28.7153, 4.1393)
  line L813 (28.7153, 4.1393) -> (28.6928, 4.0208)
  line L814 (28.6928, 4.0208) -> (28.6674, 3.912)
  line L815 (28.6674, 3.912) -> (28.6391, 3.8103)
  line L816 (28.6391, 3.8103) -> (28.6103, 3.7211)
  line L817 (28.6103, 3.7211) -> (28.5791, 3.6371)
  line L818 (28.5791, 3.6371) -> (28.5192, 3.5015)
  line L819 (28.5192, 3.5015) -> (28.4622, 3.3971)
  line L820 (28.4622, 3.3971) -> (28.4154, 3.3262)
  line L821 (28.4154, 3.3262) -> (28.3924, 3.2964)
  line L822 (28.3924, 3.2964) -> (28.2992, 3.2317)
  line L823 (28.2992, 3.2317) -> (28.2173, 3.1653)
  line L824 (28.2173, 3.1653) -> (28.1466, 3.098)
  line L825 (28.1466, 3.098) -> (28.0871, 3.0308)
  line L826 (28.0871, 3.0308) -> (28.0387, 2.9643)
  line L827 (28.0387, 2.9643) -> (28.0011, 2.8994)
  line L828 (28.0011, 2.8994) -> (27.974, 2.837)
  line L829 (27.974, 2.837) -> (27.9574, 2.7776)
  line L830 (27.9574, 2.7776) -> (27.9507, 2.7222)
  line L831 (27.9507, 2.7222) -> (27.9536, 2.6714)
  line L832 (27.9536, 2.6714) -> (27.9658, 2.6259)
  line L833 (27.9658, 2.6259) -> (27.9933, 2.5776)
  line L834 (27.9933, 2.5776) -> (28.089, 2.4617)
  line L835 (28.089, 2.4617) -> (28.1956, 2.3217)
  line L836 (28.1956, 2.3217) -> (28.2958, 2.1772)
  line L837 (28.2958, 2.1772) -> (28.3764, 2.0503)
  line L838 (28.3764, 2.0503) -> (28.4139, 2.0092)
  line L839 (28.4139, 2.0092) -> (28.4534, 1.9836)
  line L840 (28.4534, 1.9836) -> (28.5008, 1.9651)
  line L841 (28.5008, 1.9651) -> (28.5556, 1.9543)
  line L842 (28.5556, 1.9543) -> (28.6172, 1.9519)
  line L843 (28.6172, 1.9519) -> (28.6849, 1.9583)
  line L844 (28.6849, 1.9583) -> (28.7582, 1.974)
  line L845 (28.7582, 1.974) -> (28.8364, 1.9996)
  line L846 (28.8364, 1.9996) -> (28.9188, 2.0354)
  line L847 (28.9188, 2.0354) -> (29.0045, 2.0818)
  line L848 (29.0045, 2.0818) -> (29.093, 2.1392)
  line L849 (29.093, 2.1392) -> (29.1833, 2.2078)
  line L850 (29.1833, 2.2078) -> (29.2188, 2.2205)
  line L851 (29.2188, 2.2205) -> (29.3008, 2.2431)
  line L852 (29.3008, 2.2431) -> (29.4176, 2.265)
  line L853 (29.4176, 2.265) -> (29.5651, 2.2802)
  line L854 (29.5651, 2.2802) -> (29.6546, 2.2838)
  line L855 (29.6546, 2.2838) -> (29.7483, 2.2837)
  line L856 (29.7483, 2.2837) -> (29.8539, 2.2792)
  line L857 (29.8539, 2.2792) -> (29.9652, 2.2697)
  line L858 (29.9652, 2.2697) -> (30.0848, 2.2545)
  line L859 (30.0848, 2.2545) -> (30.2119, 2.2329)
  line L860 (30.2119, 2.2329) -> (30.3467, 2.2041)
  line L861 (30.3467, 2.2041) -> (30.4868, 2.1679)
  line L862 (30.4868, 2.1679) -> (30.6086, 2.1313)
  arc A17 (30.7902, 1.5727) -> (30.6086, 2.1313) centre (25, 0) ccw
  line L863 (30.7902, 1.5727) -> (30.7131, 1.4714)
  line L864 (30.7131, 1.4714) -> (30.6209, 1.3597)
  line L865 (30.6209, 1.3597) -> (30.5288, 1.2572)
  line L866 (30.5288, 1.2572) -> (30.4388, 1.165)
  line L867 (30.4388, 1.165) -> (30.3509, 1.0823)
  line L868 (30.3509, 1.0823) -> (30.2664, 1.0092)
  line L869 (30.2664, 1.0092) -> (30.1837, 0.9435)
  line L870 (30.1837, 0.9435) -> (30.108, 0.8884)
  line L871 (30.108, 0.8884) -> (30.0334, 0.8387)
  line L872 (30.0334, 0.8387) -> (29.9052, 0.7643)
  line L873 (29.9052, 0.7643) -> (29.7978, 0.7133)
  line L874 (29.7978, 0.7133) -> (29.7182, 0.6834)
  line L875 (29.7182, 0.6834) -> (29.6821, 0.6728)
  line L876 (29.6821, 0.6728) -> (29.5686, 0.6752)
  line L877 (29.5686, 0.6752) -> (29.4633, 0.6697)
  line L878 (29.4633, 0.6697) -> (29.3666, 0.6568)
  line L879 (29.3666, 0.6568) -> (29.279, 0.6373)
  line L880 (29.279, 0.6373) -> (29.2007, 0.6121)
  line L881 (29.2007, 0.6121) -> (29.1322, 0.5817)
  line L882 (29.1322, 0.5817) -> (29.0736, 0.547)
  line L883 (29.0736, 0.547) -> (29.0252, 0.5089)
  line L884 (29.0252, 0.5089) -> (28.9872, 0.4679)
  line L885 (28.9872, 0.4679) -> (28.9597, 0.4251)
  line L886 (28.9597, 0.4251) -> (28.9428, 0.3812)
  line L887 (28.9428, 0.3812) -> (28.9367, 0.3259)
  line L888 (28.9367, 0.3259) -> (28.9461, 0.1759)
  line L889 (28.9461, 0.1759) -> (28.95, 0)
  line L890 (28.95, 0) -> (28.9461, -0.1759)
  line L891 (28.9461, -0.1759) -> (28.9367, -0.3259)
  line L892 (28.9367, -0.3259) -> (28.9428, -0.3812)
  line L893 (28.9428, -0.3812) -> (28.9597, -0.4251)
  line L894 (28.9597, -0.4251) -> (28.9872, -0.468)
  line L895 (28.9872, -0.468) -> (29.0252, -0.5089)
  line L896 (29.0252, -0.5089) -> (29.0736, -0.5471)
  line L897 (29.0736, -0.5471) -> (29.1322, -0.5817)
  line L898 (29.1322, -0.5817) -> (29.2007, -0.6121)
  line L899 (29.2007, -0.6121) -> (29.279, -0.6374)
  line L900 (29.279, -0.6374) -> (29.3666, -0.6568)
  line L901 (29.3666, -0.6568) -> (29.4633, -0.6697)
  line L902 (29.4633, -0.6697) -> (29.5686, -0.6752)
  line L903 (29.5686, -0.6752) -> (29.6821, -0.6728)
  line L904 (29.6821, -0.6728) -> (29.7182, -0.6834)
  line L905 (29.7182, -0.6834) -> (29.7978, -0.7133)
  line L906 (29.7978, -0.7133) -> (29.9052, -0.7643)
  line L907 (29.9052, -0.7643) -> (30.0334, -0.8387)
  line L908 (30.0334, -0.8387) -> (30.108, -0.8884)
  line L909 (30.108, -0.8884) -> (30.1837, -0.9435)
  line L910 (30.1837, -0.9435) -> (30.2664, -1.0092)
  line L911 (30.2664, -1.0092) -> (30.3509, -1.0824)
  line L912 (30.3509, -1.0824) -> (30.4388, -1.165)
  line L913 (30.4388, -1.165) -> (30.5288, -1.2572)
  line L914 (30.5288, -1.2572) -> (30.6209, -1.3597)
  line L915 (30.6209, -1.3597) -> (30.7131, -1.4714)
  line L916 (30.7131, -1.4714) -> (30.7902, -1.5727)
  arc A18 (30.6087, -2.1311) -> (30.7902, -1.5727) centre (25, 0) ccw
  line L917 (30.6087, -2.1311) -> (30.4869, -2.1677)
  line L918 (30.4869, -2.1677) -> (30.3467, -2.2039)
  line L919 (30.3467, -2.2039) -> (30.2119, -2.2327)
  line L920 (30.2119, -2.2327) -> (30.0848, -2.2544)
  line L921 (30.0848, -2.2544) -> (29.9652, -2.2696)
  line L922 (29.9652, -2.2696) -> (29.8539, -2.2791)
  line L923 (29.8539, -2.2791) -> (29.7483, -2.2836)
  line L924 (29.7483, -2.2836) -> (29.6546, -2.2837)
  line L925 (29.6546, -2.2837) -> (29.5651, -2.2801)
  line L926 (29.5651, -2.2801) -> (29.4177, -2.265)
  line L927 (29.4177, -2.265) -> (29.3008, -2.243)
  line L928 (29.3008, -2.243) -> (29.2188, -2.2204)
  line L929 (29.2188, -2.2204) -> (29.1834, -2.2077)
  line L930 (29.1834, -2.2077) -> (29.093, -2.1391)
  line L931 (29.093, -2.1391) -> (29.0045, -2.0817)
  line L932 (29.0045, -2.0817) -> (28.9188, -2.0353)
  line L933 (28.9188, -2.0353) -> (28.8364, -1.9995)
  line L934 (28.8364, -1.9995) -> (28.7582, -1.974)
  line L935 (28.7582, -1.974) -> (28.6849, -1.9582)
  line L936 (28.6849, -1.9582) -> (28.6172, -1.9519)